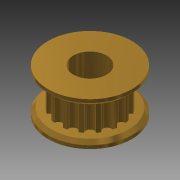
# Autodesk Inventor part: stepper_gear_28
Saved by Autodesk Inventor 2013 (Build 170138000, 138)
## iProperties
Shininess: 27.0
Created: 2013-02-12
Part Number: stepper_gear_28
Document SubType Name: Modeling
Designer: Noa Izumi
Material: Default
Density: 1 g/cm^3
Density: 0.0
Volumn: 0.0
Area: 0.0
PropertySet Name: Model Information
Control State: 0
Master: False
Checked Out: False
Author: Noa Izumi
Autodesk Inventor part; units mm, degrees
ref_plane "YZ Plane" through (0, 0, 0) normal (1, 0, 0) x (0, 1, 0)
ref_plane "XZ Plane" through (0, 0, 0) normal (0, 1, 0) x (-1, 0, 0)
ref_plane "XY Plane" through (0, 0, 0) normal (0, 0, 1) x (1, 0, 0)
sketch "Sketch1" plane through (0, 0, 0) normal (0, 0, 1) x (1, 0, 0)
  circle A0 centre (0, 0) radius 6.3
  dimension "d0" = 12.6
  constraints: 1 centre point
  measures "d0" diameter of A0
extrude "Extrusion1" add sketch "Sketch1" along normal blind 1
sketch "Sketch2" plane through (0, 0, 1) normal (0, 0, 1) x (1, 0, 0)
  circle A0 centre (0, 0) radius 6.3 projected
  circle A1 centre (0, 0) radius 4.75
  dimension "d3" = 9.5
  constraints: 1 centre point, 1 coincident
  measures "d3" diameter of A1
extrude "Extrusion2" add sketch "Sketch2" along normal blind 4.5 contours A1
sketch "Sketch3" plane through (0, 0, 5.5) normal (0, 0, 1) x (1, 0, 0)
  circle A0 centre (0, 0) radius 4.75 projected
  circle A1 centre (0, 4.75) radius 0.65
  dimension "d6" = 1.3
  constraints: 1 centre point, 1 vertical alignment, 1 other
  measures "d6" diameter of A1
extrude "Extrusion3" cut sketch "Sketch3" against normal blind 4.5 contours A1 A0 | A0 A1 picked at (-0.025, 4.5315) picked at (0.0193, 4.9625)
pattern_circular "Circular Pattern1" count 16 over 360 about axis through (0, 0, 1) along (0, 0, 1) of "Extrusion3"
sketch "Sketch4" plane through (0, 0, 5.5) normal (0, 0, 1) x (1, 0, 0)
  arc A0 (2.8688, 3.7859) -> (2.3998, 4.0992) centre (0, 0) ccw projected
  circle A1 centre (0, 0) radius 6.3
  dimension "d12" = 12.6
  constraints: 1 centre point, 1 coincident
  measures "d12" diameter of A1
extrude "Extrusion4" add sketch "Sketch4" along normal blind 1
sketch "Sketch5" plane through (0, 0, 6.5) normal (0, 0, 1) x (1, 0, 0)
  circle A0 centre (0, 0) radius 6.3 projected
  constraints: 1 coincident
hole "Hole1" at (0, 0, 6.5) direction (0, 0, -1) diameter 5 end through all
chamfer "Chamfer1" distance 0.5 angle 45 2 edges at (-6.3, 0, 5.5) (-6.3, 0, 1)
